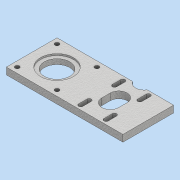
# Autodesk Inventor part: Uchwyt silnika krokowego osi X - płaski
Saved by Autodesk Inventor 2018 (Build 220112000, 112)
## iProperties
Created: 2019-01-30
Part Number: Uchwyt silnika krokowego osi X - płaski
Material: Ogólny
Document SubType Name: Modeling
Designer: Dawid
Density: 1 g/cm^3
Appearance: Aluminium odlewane
Author: Dawid
Autodesk Inventor part; units mm, degrees
ref_plane "YZ Plane" through (0, 0, 0) normal (1, 0, 0) x (0, 1, 0)
ref_plane "XZ Plane" through (0, 0, 0) normal (0, 1, 0) x (-1, 0, 0)
ref_plane "XY Plane" through (0, 0, 0) normal (0, 0, 1) x (1, 0, 0)
sketch "Szkic1" plane through (0, 0, 0) normal (0, 0, 1) x (1, 0, 0)
  arc A0 (89.3398, 60) -> (106.6602, 60) centre (98, 65.0001) ccw
  line L0 (70, 60) -> (89.3398, 60)
  line L1 (70, 0) -> (70, 60)
  line L2 (70, 0) -> (138, 0)
  line L3 (138, 60) -> (138, 0)
  line L4 (106.6602, 60) -> (138, 60)
  line L5 (80.5, 5) -> (80.5, 15)
  arc A1 (85.5, 15) -> (80.5, 15) centre (83, 15) ccw
  line L6 (85.5, 15) -> (85.5, 5)
  arc A2 (80.5, 5) -> (85.5, 5) centre (83, 5) ccw
  line L7 (115.5, 55) -> (115.5, 45)
  arc A3 (110.5, 45) -> (115.5, 45) centre (113, 45) ccw
  line L8 (110.5, 45) -> (110.5, 55)
  arc A4 (115.5, 55) -> (110.5, 55) centre (113, 55) ccw
  line L9 (80.5, 45) -> (80.5, 55)
  arc A5 (85.5, 55) -> (80.5, 55) centre (83, 55) ccw
  line L10 (85.5, 55) -> (85.5, 45)
  arc A6 (80.5, 45) -> (85.5, 45) centre (83, 45) ccw
  line L11 (115.5, 15) -> (115.5, 5)
  arc A7 (110.5, 5) -> (115.5, 5) centre (113, 5) ccw
  line L12 (110.5, 5) -> (110.5, 15)
  arc A8 (115.5, 15) -> (110.5, 15) centre (113, 15) ccw
  line L13 (88, 25) -> (88, 35)
  arc A9 (108, 35) -> (88, 35) centre (98, 35) ccw
  line L14 (108, 35) -> (108, 25)
  arc A10 (88, 25) -> (108, 25) centre (98, 25) ccw
  circle A11 centre (30, 30) radius 19.5
  circle A12 centre (53.57, 53.57) radius 2.5
  circle A13 centre (6.43, 6.43) radius 2.5
  circle A14 centre (6.43, 53.57) radius 2.5
  circle A15 centre (53.57, 6.43) radius 2.5
  line L15 (70, 60) -> (70, 0)
  line L16 (0, 60) -> (70, 60)
  line L17 (0, 0) -> (0, 60)
  line L18 (70, 0) -> (0, 0)
  circle A16 centre (30, 30) radius 15
  point P0 (35, 30)
  constraints: 38 end point, 22 point on circle, 17 centre point
extrude "Wyciągnięcie proste1" add sketch "Szkic1" along normal blind 8 contours A0 L4 L3 L2 L1 L0 | L1 L18 L17 L16
sketch "Szkic2" plane through (0, 0, 0) normal (0, 0, -1) x (-1, 0, 0)
  circle A0 centre (-30, 30) radius 15 projected
  circle A1 centre (-30, 30) radius 19.5 projected
  point P0 (0, 0)
extrude "Wyciągnięcie proste2" add sketch "Szkic2" against normal blind 6
thread "Gwint1" size "M5x0.8" class "6H" standard "ANSI Metric M Profile" full length
thread "Gwint2" size "M5x0.8" class "6H" standard "ANSI Metric M Profile" full length
thread "Gwint3" size "M5x0.8" class "6H" standard "ANSI Metric M Profile" full length
thread "Gwint4" size "M5x0.8" class "6H" standard "ANSI Metric M Profile" full length
